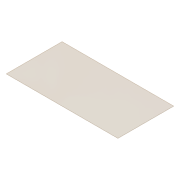
# Autodesk Inventor part: BottomLexan
Saved by Autodesk Inventor 2012 (Build 160160000, 160)
## iProperties
Created: 2013-01-14
Part Number: BottomLexan
Material: Polycarbonate, Smoke
Document SubType Name: Modeling
Designer: JesseK
Density: 1.2 g/cm^3
Mass: 324.464 g
Surface Area: 3434.67 cm^2
Volume: 270.387 cm^3
Author: JesseK
Autodesk Inventor part; units mm, degrees
ref_plane "YZ Plane" through (0, 0, 0) normal (1, 0, 0) x (0, 1, 0)
ref_plane "XZ Plane" through (0, 0, 0) normal (0, 1, 0) x (-1, 0, 0)
ref_plane "XY Plane" through (0, 0, 0) normal (0, 0, 1) x (1, 0, 0)
sketch "Sketch2" plane through (0, 0, 0) normal (0, 1, 0) x (-1, 0, 0)
  line L0 (0, 0) -> (0, -304.8)
  line L1 (0, -304.8) -> (609.6, -304.8)
  line L2 (609.6, -304.8) -> (609.6, 0)
  line L3 (609.6, 0) -> (0, 0)
  point P0 (0, 0)
  dimension "d0" = 609.6
  dimension "d1" = 304.8
  constraints: 8 end point, 2 horizontal, 2 vertical, 1 coincident, 1 parallel
  measures "d0" distance of L2.end L0.start
  measures "d1" distance of L0.end point (0, 0)
extrude "Extrusion1" add sketch "Sketch2" along normal blind 1.5875
body "Solid1"
